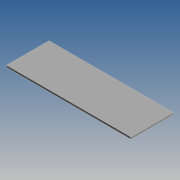
# Autodesk Inventor part: F115Reseau
Saved by Autodesk Inventor 2015 SP1 (Build 190203100, 203)
## iProperties
Created: 2017-05-18
Part Number: F115Reseau
Material: Générique
Document SubType Name: Modeling
Designer: serge.amoos
Density: 1 g/cm^3
Appearance: Par défaut
Author: serge.amoos
Autodesk Inventor part; units mm, degrees
ref_plane "YZ Plane" through (0, 0, 0) normal (1, 0, 0) x (0, 1, 0)
ref_plane "XZ Plane" through (0, 0, 0) normal (0, 1, 0) x (-1, 0, 0)
ref_plane "XY Plane" through (0, 0, 0) normal (0, 0, 1) x (1, 0, 0)
sketch "Sketch1" plane through (0, 0, 0) normal (0, 0, 1) x (1, 0, 0)
  line L0 (-53.34, 0) -> (53.34, 0) construction
  line L1 (0, -18.2) -> (0, 18.2) construction
  line L2 (-38.1, 13) -> (38.1, 13)
  line L3 (38.1, 13) -> (38.1, -13)
  line L4 (38.1, -13) -> (-38.1, -13)
  line L5 (-38.1, -13) -> (-38.1, 13)
  point P0 (0, 0)
  point P1 (0, 13)
  point P2 (-38.1, 0)
  dimension "d0" = 76.2
  dimension "d1" = 26
  constraints: 8 end point, 2 midpoint, 2 parallel, 2 point on line, 1 horizontal, 1 perpendicular
  measures "d0" distance of L2.start L2.end
  measures "d1" distance of L4.end L2.start
extrude "Extrusion1" add sketch "Sketch1" along normal blind 1.2
body "Solid1"
